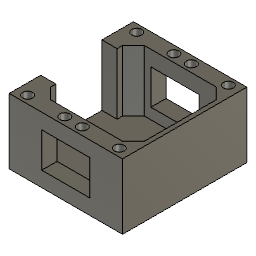
モーター支え(下)(左) (Autodesk Fusion 360 design; units mm, degrees)
Autodesk Fusion 360 part; units mm, degrees
note: some values were not read from the file. Set by a fixed rule: which sketch regions a step uses.
sketch "スケッチ1" plane through (0, 0, 0) normal (0, 0, 1) x (1, 0, 0)
  line L0 (0, 0) -> (52, 0)
  line L1 (52, 0) -> (52, 57)
  line L2 (52, 57) -> (0, 57)
  line L3 (0, 57) -> (0, 0)
  dimension "d1" = 57
  constraint horizontal L0
  constraint vertical L1
  constraint horizontal L2
  constraint vertical L3
  constraint coincident L0.start L3.end
  measures "d1" distance of L0.start L2.end
extrude "押し出し1" add sketch "スケッチ1" along normal blind 30
sketch "スケッチ2" plane through (0, 0, 30) normal (0, 0, 1) x (-1, 0, 0)
  line L0 (0, -57) -> (0, 0)
  line L1 (0, 0) -> (-52, 0)
  line L2 (-52, 0) -> (-52, -57)
  line L3 (-52, -57) -> (0, -57)
  line L4 (-45, -7) -> (-45, -50)
  line L5 (-45, -50) -> (-7, -50)
  line L6 (-7, -50) -> (-7, -7)
  line L7 (-12, -7) -> (-45, -7)
  line L8 (-45, -7) -> (-50, -7)
  line L9 (-50, -12) -> (-50, -50)
  line L10 (-50, -50) -> (-45, -50)
  line L11 (-45, -50) -> (-45, -7)
  line L12 (-7, -7) -> (-45, -7)
  line L13 (-50, -7) -> (-50, -45)
  line L14 (-45, -50) -> (-12, -50)
  line L15 (-7, -45) -> (-7, -12)
  line L16 (-7, -45) -> (-12, -50)
  line L17 (-45, -50) -> (-50, -45)
  line L18 (-45, -7) -> (-50, -12)
  line L19 (-12, -7) -> (-7, -12)
  point P0 (-7, -50)
  dimension "d5" = 5
  dimension "d6" = 5
  dimension "d7" = 5
  dimension "d8" = 5
  dimension "d9" = 5
  dimension "d10" = 5
  dimension "d11" = 5
  dimension "d12" = 5
  constraint horizontal L8
  constraint vertical L9
  constraint horizontal L10
  constraint vertical L11
  constraint horizontal L12
  constraint vertical L13
  constraint horizontal L14
  constraint vertical L15
  constraint coincident P0 L15
  constraint coincident P0 L14
  constraint coincident L9.end L14
  constraint coincident L9.end L13
  constraint coincident L8.end L12
  constraint coincident L8.end L9
  constraint coincident L6.end L7
  constraint coincident L6.end L15
  measures "d5" distance of P0 L15.start
  measures "d6" distance of P0 L14.end
  measures "d7" distance of L9.end L4.end
  measures "d8" distance of L9.end L13.end
  measures "d9" distance of L8.end L4.start
  measures "d10" distance of L8.end L9.start
  measures "d11" distance of L6.end L7.start
  measures "d12" distance of L6.end L15.end
extrude "押し出し2" cut sketch "スケッチ2" against normal blind 28 contours L4 L5 L6 L7 L11 L12 L14 L15 L16 L19 | L4 L9 L11 L13 L17 L18
sketch "スケッチ3" plane through (0, 0, 30) normal (0, 0, 1) x (-1, 0, 0)
  line L0 (-50, -45) -> (-50, -12)
  line L1 (-50, -12) -> (-45, -7)
  line L2 (-45, -7) -> (-12, -7)
  line L3 (-12, -7) -> (-7, -12)
  line L4 (-7, -12) -> (-7, -45)
  line L5 (-7, -45) -> (-12, -50)
  line L6 (-12, -50) -> (-45, -50)
  line L7 (-45, -50) -> (-50, -45)
  line L8 (0, -57) -> (0, 0)
  line L9 (0, 0) -> (-52, 0)
  line L10 (-52, 0) -> (-52, -57)
  line L11 (-52, -57) -> (0, -57)
  line L12 (0, -57) -> (-26.0227, -57)
  line L13 (-26.0227, -57) -> (-26.0227, -53.5)
  line L14 (-26.0227, -53.5) -> (0, -53.5)
  line L15 (0, -53.5) -> (0, -57)
  line L16 (-26.0227, -53.5) -> (-52, -53.5)
  line L17 (-52, -53.5) -> (-52, -57)
  line L18 (-52, -57) -> (-26.0227, -57)
  line L19 (-26.0227, -57) -> (-26.0227, -53.5)
  line L20 (0, 0) -> (-26.0083, 0)
  line L21 (-26.0083, 0) -> (-26.0083, -3.5)
  line L22 (-26.0083, -3.5) -> (0, -3.5)
  line L23 (0, -3.5) -> (0, 0)
  line L24 (-26.0083, 0) -> (-52, 0)
  line L25 (-52, 0) -> (-52, -3.5)
  line L26 (-52, -3.5) -> (-26.0083, -3.5)
  line L27 (-26.0083, -3.5) -> (-26.0083, 0)
  line L28 (0, -57) -> (-5, -57)
  line L29 (-5, -57) -> (-5, -53.5)
  line L30 (-5, -53.5) -> (0, -53.5)
  line L31 (0, -53.5) -> (0, -57)
  line L32 (-52, -57) -> (-47, -57)
  line L33 (-47, -57) -> (-47, -53.5)
  line L34 (-47, -53.5) -> (-52, -53.5)
  line L35 (-52, -53.5) -> (-52, -57)
  line L36 (0, 0) -> (-5, 0)
  line L37 (-5, 0) -> (-5, -3.5)
  line L38 (-5, -3.5) -> (0, -3.5)
  line L39 (0, -3.5) -> (0, 0)
  line L40 (-52, 0) -> (-47, 0)
  line L41 (-47, 0) -> (-47, -3.5)
  line L42 (-47, -3.5) -> (-52, -3.5)
  line L43 (-52, -3.5) -> (-52, 0)
  line L44 (-26.0227, -53.5) -> (-30.042, -53.5)
  line L45 (-30.042, -53.5) -> (-30.042, -57)
  line L46 (-30.042, -57) -> (-26.0227, -57)
  line L47 (-26.0227, -57) -> (-26.0227, -53.5)
  line L48 (-26.0227, -53.5) -> (-22.0467, -53.5)
  line L49 (-22.0467, -53.5) -> (-22.0467, -57)
  line L50 (-22.0467, -57) -> (-26.0227, -57)
  line L51 (-26.0227, -57) -> (-26.0227, -53.5)
  line L52 (-26.0083, 0) -> (-30.0469, 0)
  line L53 (-30.0469, 0) -> (-30.0469, -3.5)
  line L54 (-30.0469, -3.5) -> (-26.0083, -3.5)
  line L55 (-26.0083, -3.5) -> (-26.0083, 0)
  line L56 (-26.0083, 0) -> (-22.0451, 0)
  line L57 (-22.0451, 0) -> (-22.0451, -3.5)
  line L58 (-22.0451, -3.5) -> (-26.0083, -3.5)
  line L59 (-26.0083, -3.5) -> (-26.0083, 0)
  circle A0 centre (-5, -53.5) radius 2.25
  circle A1 centre (-22.0467, -53.5) radius 2.25
  circle A2 centre (-30.042, -53.5) radius 2.25
  circle A3 centre (-47, -53.5) radius 2.25
  circle A4 centre (-5, -3.5) radius 2.25
  circle A5 centre (-22.0451, -3.5) radius 2.25
  circle A6 centre (-30.0469, -3.5) radius 2.25
  circle A7 centre (-47, -3.5) radius 2.25
  dimension "d15" = 3.5
  dimension "d16" = 3.5
  dimension "d17" = 3.5
  dimension "d18" = 4.5
  dimension "d19" = 4.5
  dimension "d20" = 4.5
  dimension "d21" = 4.5
  dimension "d22" = 4.5
  dimension "d23" = 4.5
  dimension "d24" = 4.5
  dimension "d25" = 4.5
  constraint horizontal L12
  constraint vertical L13
  constraint horizontal L14
  constraint vertical L15
  constraint coincident L8.start L11.end
  constraint horizontal L16
  constraint vertical L17
  constraint horizontal L18
  constraint vertical L19
  constraint coincident L10.end L11.start
  constraint horizontal L20
  constraint vertical L21
  constraint horizontal L22
  constraint vertical L23
  constraint coincident L8.end L9.start
  constraint horizontal L24
  constraint vertical L25
  constraint horizontal L26
  constraint vertical L27
  constraint horizontal L28
  constraint vertical L29
  constraint horizontal L30
  constraint vertical L31
  constraint coincident L14 L29.end
  constraint horizontal L32
  constraint vertical L33
  constraint horizontal L34
  constraint vertical L35
  constraint coincident L16 L33.end
  constraint horizontal L36
  constraint vertical L37
  constraint horizontal L38
  constraint vertical L39
  constraint coincident L22 L37.end
  constraint horizontal L40
  constraint vertical L41
  constraint horizontal L42
  constraint vertical L43
  constraint coincident L26 L41.end
  constraint horizontal L44
  constraint vertical L45
  constraint horizontal L46
  constraint vertical L47
  constraint coincident L11 L45.end
  constraint horizontal L48
  constraint vertical L49
  constraint horizontal L50
  constraint vertical L51
  constraint coincident L12 L49.end
  constraint horizontal L52
  constraint vertical L53
  constraint horizontal L54
  constraint vertical L55
  constraint coincident L26 L53.end
  constraint horizontal L56
  constraint vertical L57
  constraint horizontal L58
  constraint vertical L59
  constraint coincident L22 L57.end
  constraint coincident L29.end L30.start
  constraint coincident L48.end L49.start
  constraint coincident L44.end L45.start
  constraint coincident L33.end L34.start
  constraint coincident L37.end L38.start
  constraint coincident L57.end L58.start
  constraint coincident L53.end L54.start
  constraint coincident L41.end L42.start
  measures "d15" distance of L8.start L14.end
  measures "d16" distance of L8.end L22.end
  measures "d17" distance of L20.end L21.end
  measures "d18" diameter of A0
  measures "d19" diameter of A1
  measures "d20" diameter of A2
  measures "d21" diameter of A3
  measures "d22" diameter of A4
  measures "d23" diameter of A5
  measures "d24" diameter of A6
  measures "d25" diameter of A7
extrude "押し出し3" cut sketch "スケッチ3" against normal blind 6 contours L14 L29 L30 A0 | L14 L30 A0 | L14 L29 A0 | L22 L38 A4 | L22 L37 L38 A4 | L14 L48 L49 A1 | L14 L49 A1 | L22 L37 A4 | L14 L48 A1 | L22 L58 A5 | L22 L57 A5 | L16 L45 A2 | L16 L44 L45 A2 | L16 L44 A2 | L22 L57 L58 A5 | L16 L33 L34 A3 | L16 L33 A3 | L16 L34 A3 | L26 L53 L54 A6 | L26 L53 A6 | L26 L54 A6 | L26 L41 A7 | L26 L41 L42 A7 | L26 L42 A7
sketch "スケッチ4" plane through (0, 0, 24) normal (0, 0, 1) x (-1, 0, 0)
  circle A0 centre (-5, -53.5) radius 2.25
  circle A1 centre (-5, -53.5) radius 1.65
  circle A2 centre (-5, -3.5) radius 1.65
  circle A3 centre (-47, -3.5) radius 1.65
  circle A4 centre (-47, -53.5) radius 1.65
  dimension "d28" = 3.3
  dimension "d29" = 3.3
  dimension "d30" = 3.3
  dimension "d31" = 3.3
  constraint concentric A0 A1
  measures "d28" diameter of A1
  measures "d29" diameter of A2
  measures "d30" diameter of A3
  measures "d31" diameter of A4
extrude "押し出し4" cut sketch "スケッチ4" against normal blind 24 contours A1 | A2 | A3 | A4
sketch "スケッチ5" plane through (0, 0, 0) normal (-1, 0, 0) x (0, -1, 0)
  line L0 (-57, 0) -> (0, 0)
  line L1 (0, 0) -> (0, 30)
  line L2 (0, 30) -> (-57, 30)
  line L3 (-57, 30) -> (-57, 0)
  line L4 (-57, 0) -> (-28.5, 0)
  line L5 (-28.5, 0) -> (-28.5, 2)
  line L6 (-28.5, 2) -> (-57, 2)
  line L7 (-57, 2) -> (-57, 0)
  line L8 (-28.5, 2) -> (-14.5, 2)
  line L9 (-14.5, 2) -> (-14.5, 30)
  line L10 (-14.5, 30) -> (-28.5, 30)
  line L11 (-28.5, 30) -> (-28.5, 2)
  line L12 (-28.5, 2) -> (-42.5, 2)
  line L13 (-42.5, 2) -> (-42.5, 30)
  line L14 (-42.5, 30) -> (-28.5, 30)
  line L15 (-28.5, 30) -> (-28.5, 2)
  dimension "d34" = 28.5
  dimension "d35" = 2
  dimension "d36" = 14
  dimension "d37" = 28
  dimension "d38" = 14
  dimension "d39" = 28
  constraint horizontal L4
  constraint vertical L5
  constraint horizontal L6
  constraint vertical L7
  constraint coincident L0.start L3.end
  constraint horizontal L8
  constraint vertical L9
  constraint horizontal L10
  constraint vertical L11
  constraint horizontal L12
  constraint vertical L13
  constraint horizontal L14
  constraint vertical L15
  measures "d34" distance of L0.start L4.end
  measures "d35" distance of L0.start L6.end
  measures "d36" distance of L5.end L8.end
  measures "d37" distance of L5.end L10.end
  measures "d38" distance of L5.end L12.end
  measures "d39" distance of L5.end L10.end
extrude "押し出し5" cut sketch "スケッチ5" against normal blind 7 contours L2 L8 L9 L10 L11 L15 | L2 L6 L11 L12 L13 L14 L15
sketch "スケッチ6" plane through (0, 0, 0) normal (0, -1, 0) x (1, 0, 0)
  line L0 (0, 0) -> (52, 0)
  line L1 (52, 0) -> (52, 30)
  line L2 (52, 30) -> (0, 30)
  line L3 (0, 30) -> (0, 0)
  line L4 (0, 30) -> (15, 30)
  line L5 (15, 30) -> (15, 0)
  line L6 (15, 0) -> (0, 0)
  line L7 (0, 0) -> (0, 30)
  line L8 (52, 0) -> (37, 0)
  line L9 (37, 0) -> (37, 30)
  line L10 (37, 30) -> (52, 30)
  line L11 (52, 30) -> (52, 0)
  line L12 (0, 30) -> (52, 30)
  line L13 (52, 30) -> (52, 23)
  line L14 (52, 23) -> (0, 23)
  line L15 (0, 23) -> (0, 30)
  line L16 (0, 0) -> (52, 0)
  line L17 (52, 0) -> (52, 7)
  line L18 (52, 7) -> (0, 7)
  line L19 (0, 7) -> (0, 0)
  dimension "d42" = 15
  dimension "d43" = 30
  dimension "d44" = 15
  dimension "d45" = 30
  dimension "d46" = 7
  dimension "d47" = 7
  constraint horizontal L4
  constraint vertical L5
  constraint horizontal L6
  constraint vertical L7
  constraint coincident L2.end L3.start
  constraint horizontal L8
  constraint vertical L9
  constraint horizontal L10
  constraint vertical L11
  constraint coincident L0.end L1.start
  constraint horizontal L12
  constraint vertical L13
  constraint horizontal L14
  constraint vertical L15
  constraint horizontal L16
  constraint vertical L17
  constraint horizontal L18
  constraint vertical L19
  constraint coincident L0.start L3.end
  measures "d42" distance of L2.end L4.end
  measures "d43" distance of L2.end L0.start
  measures "d44" distance of L0.end L8.end
  measures "d45" distance of L0.end L1.end
  measures "d46" distance of L2.end L14.end
  measures "d47" distance of L0.start L18.end
extrude "押し出し6" cut sketch "スケッチ6" against normal blind 7 contours L5 L9 L14 L18
sketch "スケッチ7" plane through (0, 57, 0) normal (0, 1, 0) x (-1, 0, 0)
  line L0 (-52, 0) -> (0, 0)
  line L1 (0, 0) -> (0, 30)
  line L2 (0, 30) -> (-52, 30)
  line L3 (-52, 30) -> (-52, 0)
  line L4 (-52, 0) -> (-37, 0)
  line L5 (-37, 0) -> (-37, 30)
  line L6 (-37, 30) -> (-52, 30)
  line L7 (-52, 30) -> (-52, 0)
  line L8 (0, 0) -> (-15, 0)
  line L9 (-15, 0) -> (-15, 30)
  line L10 (-15, 30) -> (0, 30)
  line L11 (0, 30) -> (0, 0)
  line L12 (-52, 30) -> (0, 30)
  line L13 (0, 30) -> (0, 23)
  line L14 (0, 23) -> (-52, 23)
  line L15 (-52, 23) -> (-52, 30)
  line L16 (-52, 0) -> (0, 0)
  line L17 (0, 0) -> (0, 7)
  line L18 (0, 7) -> (-52, 7)
  line L19 (-52, 7) -> (-52, 0)
  dimension "d50" = 15
  dimension "d51" = 30
  dimension "d52" = 15
  dimension "d53" = 30
  dimension "d54" = 7
  dimension "d55" = 7
  constraint horizontal L4
  constraint vertical L5
  constraint horizontal L6
  constraint vertical L7
  constraint coincident L0.start L3.end
  constraint horizontal L8
  constraint vertical L9
  constraint horizontal L10
  constraint vertical L11
  constraint coincident L0.end L1.start
  constraint horizontal L12
  constraint vertical L13
  constraint horizontal L14
  constraint vertical L15
  constraint coincident L2.end L3.start
  constraint horizontal L16
  constraint vertical L17
  constraint horizontal L18
  constraint vertical L19
  measures "d50" distance of L0.start L4.end
  measures "d51" distance of L0.start L2.end
  measures "d52" distance of L0.end L8.end
  measures "d53" distance of L0.end L1.end
  measures "d54" distance of L2.end L14.end
  measures "d55" distance of L0.start L18.end
extrude "押し出し7" cut sketch "スケッチ7" against normal blind 7 contours L5 L9 L14 L18
equation "d6 = d5"
equation "d8 = d7"
equation "d10 = d9"
equation "d12 = d11"
